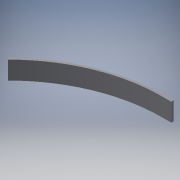
# Autodesk Inventor part: rail
Saved by Autodesk Inventor 2016 (Build 200138000, 138)
## iProperties
Created: 2016-01-16
Part Number: rail
Material: Generic
Document SubType Name: Modeling
Designer: Thariq
Density: 1 g/cm^3
Appearance: Default
Author: Thariq
Autodesk Inventor part; units mm, degrees
ref_plane "YZ Plane" through (0, 0, 0) normal (1, 0, 0) x (0, 1, 0)
ref_plane "XZ Plane" through (0, 0, 0) normal (0, 1, 0) x (-1, 0, 0)
ref_plane "XY Plane" through (0, 0, 0) normal (0, 0, 1) x (1, 0, 0)
sketch "Sketch1" plane through (0, 0, 0) normal (0, 1, 0) x (-1, 0, 0)
  arc A0 (0, -219.075) -> (154.9094, -154.9094) centre (0, 0) ccw
  arc A1 (0, -215.9) -> (152.6644, -152.6644) centre (0, 0) ccw
  line L0 (0, -215.9) -> (0, -219.075)
  line L1 (0, 0) -> (154.9094, -154.9094)
  line L2 (0, 0) -> (0, -215.9) construction
  dimension "d0" = 3.175
  dimension "d1" = 431.8
  dimension "d6" = 45
  constraints: 6 end point, 4 point on circle, 2 centre point, 2 coincident, 1 point on line, 1 vertical
  measures "d0" radial gap between concentric circles of A0 A1
  measures "d1" diameter of A1
  measures "d6" angle of L2 L1
extrude "Extrusion1" add sketch "Sketch1" along normal blind 25.4
sketch "Sketch2" plane through (0, 0, -215.9) normal (1, 0, 0) x (0, 0, -1)
  line L0 (0, 0) -> (0, 25.4) projected
  line L1 (3.175, 0) -> (3.175, 25.4) projected
  line L2 (0, 0) -> (3.175, 0)
  line L3 (3.175, 0) -> (3.175, 25.4)
  line L4 (3.175, 25.4) -> (0, 25.4)
  line L5 (0, 25.4) -> (0, 0)
  point P0 (-215.9, 0)
  constraints: 8 end point, 2 parallel, 1 horizontal, 1 perpendicular
extrude "Extrusion2" add sketch "Sketch2" along normal blind 12.7
body "Solid1"
